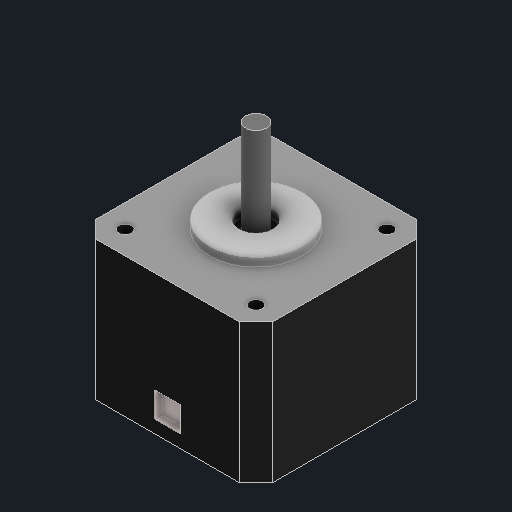
# Autodesk Inventor part: NEMA17 Stepper Motor
Saved by Autodesk Inventor 2025.1 (Build 291241000, 241)
## iProperties
Created: 2024-10-02
Part Number: NEMA17 Stepper Motor
Material: Generic
Document SubType Name: Modeling
Designer: jerem
Density: 1 g/cm^3
Appearance: Default
Author: jerem
Autodesk Inventor part; units mm, degrees
ref_plane "YZ Plane" through (0, 0, 0) normal (1, 0, 0) x (0, 1, 0)
ref_plane "XZ Plane" through (0, 0, 0) normal (0, 1, 0) x (-1, 0, 0)
ref_plane "XY Plane" through (0, 0, 0) normal (0, 0, 1) x (1, 0, 0)
sketch "Sketch1" plane through (0, 0, 0) normal (0, 1, 0) x (-1, 0, 0)
  circle A0 centre (15.5, 15.5) radius 1.5
  circle A1 centre (15.5, -15.5) radius 1.5
  circle A2 centre (-15.5, -15.5) radius 1.5
  circle A3 centre (-15.5, 15.5) radius 1.5
  circle A4 centre (0, 0) radius 11
  circle A5 centre (0, 0) radius 4
  line L0 (21, -17) -> (17, -21)
  line L1 (21, 17) -> (17, 21)
  line L2 (-17, -21) -> (-21, -17)
  line L3 (-21, 17) -> (-17, 21)
  circle A6 centre (0, 0) radius 2.5
  line L4 (17, -21) -> (-17, -21)
  line L5 (-21, -17) -> (-21, 17)
  line L6 (-17, 21) -> (17, 21)
  line L7 (21, 17) -> (21, -17)
  line L8 (0, -15.5) -> (-15.5, -15.5) construction
  line L9 (0, -15.5) -> (15.5, -15.5) construction
  line L10 (15.5, -15.5) -> (15.5, 15.5) construction
  line L11 (-15.5, -15.5) -> (-15.5, 15.5) construction
  line L12 (0, -21) -> (0, 0) construction
  line L13 (0, 0) -> (21, 0) construction
  dimension "d1" = 31
  dimension "d2" = 31
  dimension "d3" = 31
  dimension "d4" = 31
  dimension "d5" = 3
  dimension "d6" = 3
  dimension "d7" = 3
  dimension "d8" = 3
  dimension "d11" = 22
  dimension "d14" = 8
  dimension "d32" = 5
  dimension "d37" = 15.5
  dimension "d38" = 42
  dimension "d39" = 42
  dimension "d40" = 15.5
  dimension "d41" = 21
  dimension "d42" = 21
  dimension "d43" = 34
  dimension "d44" = 34
  dimension "d45" = 135
  constraints: 29 end point, 7 centre point, 6 perpendicular, 3 coincident, 3 equal length, 2 horizontal, 2 midpoint, 1 collinear, 1 vertical
  measures "d1" distance of L9.end L10.end
  measures "d2" distance of L8.end L9.end
  measures "d3" distance of L11.end L8.end
  measures "d4" distance of L10.end L11.end
  measures "d5" diameter of A0
  measures "d6" diameter of A1
  measures "d7" diameter of A2
  measures "d8" diameter of A3
  measures "d11" diameter of A4
  measures "d14" diameter of A5
  measures "d32" diameter of A6
  measures "d37" distance of L12.end L8.start
  measures "d38" distance between parallel lines of L5 L7
  measures "d39" distance between parallel lines of L6 L4
  measures "d40" distance from line of point (0, 0) L9
  measures "d41" distance of L12.start L12.end
  measures "d42" distance of L12.end L13.end
  measures "d43" distance of L1.start L0.start
  measures "d44" distance of L0.end L2.start
  measures "d45" angle of L6 L1
extrude "Extrusion1" add sketch "Sketch1" along normal blind 33 contours A4 | A5 | L0 L4 L2 L5 L3 L6 L1 L7 | A6
extrude "Extrusion2" add sketch "Sketch1" along normal blind 2 from surface at 33 contours A4 | A5 | A6
extrude "Extrusion3" cut sketch "Sketch1" against normal blind 2 from surface at 35 contours A5 | A6
sketch "Sketch2" plane through (-21, 0, 21) normal (0, 0, 1) x (1, 0, 0)
  line L0 (24, 9) -> (18, 9)
  line L1 (18, 9) -> (18, 3)
  line L2 (18, 3) -> (24, 3)
  line L3 (24, 3) -> (24, 9)
  line L4 (24, 9) -> (18, 3) construction
  line L5 (18, 9) -> (24, 3) construction
  line L6 (-8.4, 0) -> (50.4, 0) projected
  line L7 (21, -6.6) -> (21, 39.6) projected
  point P0 (21, 6)
  dimension "d17" = 6
  dimension "d18" = 6
  dimension "d46" = 3
  constraints: 12 end point, 2 midpoint, 2 parallel, 1 horizontal, 1 perpendicular, 1 point on line
  measures "d17" distance of L2.end L1.end
  measures "d18" distance of L1.end L0.end
  measures "d46" distance between parallel lines of L2 L6
extrude "Extrusion4" cut sketch "Sketch2" against normal blind 2
extrude "Extrusion5" add sketch "Sketch1" along normal blind 20 and the other way blind 2 from surface at 35 contours A6
equation "\"d2\" = d1"
equation "\"d3\" = d1"
equation "\"d4\" = d1"
equation "\"d6\" = d5"
equation "\"d7\" = d5"
equation "\"d8\" = d5"
equation "\"d37\" = 0.5 * d1"
equation "\"d39\" = d38"
equation "\"d40\" = 0.5 * d1"
equation "\"d41\" = 0.5 * d38"
equation "\"d42\" = 0.5 * d39"
body "Solid1"
